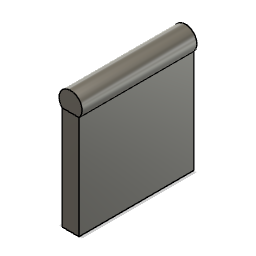
key_peg (Autodesk Fusion 360 design; units mm, degrees)
Autodesk Fusion 360 part; units mm, degrees
sketch "Sketch1" plane through (0, 0, 0) normal (0, 0, 1) x (1, 0, 0)
  circle A0 centre (0, 0) radius 3
  line L0 (0, 0) -> (-29, 0)
  line L1 (-29, 0) -> (-29, 2.2)
  line L2 (-29, 2.2) -> (0, 2.2)
  line L3 (0, 2.2) -> (0, 0)
  line L4 (0, 0) -> (-29, 0)
  line L5 (-29, 0) -> (-29, -2.2)
  line L6 (-29, -2.2) -> (0, -2.2)
  line L7 (0, -2.2) -> (0, 0)
  constraint coincident A0.centre L0.start
  constraint horizontal L0
  constraint vertical L1
  constraint horizontal L2
  constraint vertical L3
  constraint horizontal L4
  constraint vertical L5
  constraint horizontal L6
  constraint vertical L7
  constraint equal L1 L5
  constraint equal L2 L6
extrude "Extrude1" add sketch "Sketch1" along normal blind 30 makes body 1
move_body "Move1" bodies 1 to x (0, 1, 0) y (-1, 0, 0) z (0, 0, 1) at (0, 0, 0)
ref_plane "WorkPlane1" through (-2.2, -2.0396, 0) normal (0, -1, 0) x (1, 0, 0)
split "Split1" by plane through (-2.2, -2.0396, 0) normal (0, -1, 0) bodies 1 makes body 2 at (2.2, -20.0132, 10)
equation "d1 = 2 * 3 mm"
equation "d2 = 2 * 2.2 mm"
